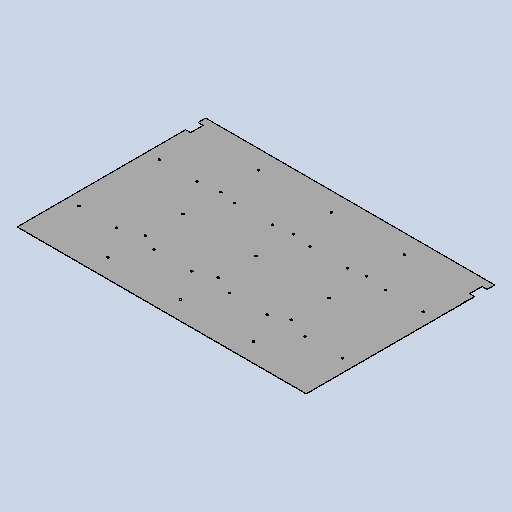
# Autodesk Inventor part: GnG L.4 floor sheet
Saved by Autodesk Inventor 2025.3 (Build 293356030, 356C)
## iProperties
Created: 2025-10-28
Part Number: GnG L.4 floor sheet
Material: Stainless Steel
Document SubType Name: Sheet Metal
Designer: admin
Mass: 82475.1 g
Surface Area: 69006.6 cm^2
Volume: 10309.4 cm^3
Density: 8 g/cm^3
Sheet Metal Rule: AISI304 3mm Die 32
Sheet Metal Width: 2300,000 mm
Sheet Metal Length: 1500,000 mm
Sheet Metal Area: 3450000,000 mm^2
Appearance: Default
Stock Number: L 4
Flat Pattern Width: 230 cm
Flat Pattern Length: 150 cm
Flat Pattern Area: 34500 cm^2
Author: admin
Autodesk Inventor part; units mm, degrees
ref_plane "YZ Plane" through (0, 0, 0) normal (1, 0, 0) x (0, 1, 0)
ref_plane "XZ Plane" through (0, 0, 0) normal (0, 1, 0) x (-1, 0, 0)
ref_plane "XY Plane" through (0, 0, 0) normal (0, 0, 1) x (1, 0, 0)
sketch "Sketch1" plane through (0, 0, 0) normal (0, 0, 1) x (1, 0, 0)
  line L0 (0, 0) -> (-2300, 0)
  line L1 (-2300, 0) -> (-2300, -1500)
  line L2 (-2300, -1500) -> (0, -1500)
  line L3 (0, -1500) -> (0, 0)
  line L4 (0, 0) -> (-20, 0)
  line L5 (-20, 0) -> (-20, -20)
  line L6 (-20, -20) -> (0, -20)
  line L7 (0, -20) -> (0, 0)
  line L8 (0, -1500) -> (-20, -1500)
  line L9 (-20, -1500) -> (-20, -1480)
  line L10 (-20, -1480) -> (0, -1480)
  line L11 (0, -1480) -> (0, -1500)
  line L12 (-2300, 0) -> (-2280, 0)
  line L13 (-2280, 0) -> (-2280, -20)
  line L14 (-2280, -20) -> (-2300, -20)
  line L15 (-2300, -20) -> (-2300, 0)
  line L16 (-2300, -1500) -> (-2280, -1500)
  line L17 (-2280, -1500) -> (-2280, -1480)
  line L18 (-2280, -1480) -> (-2300, -1480)
  line L19 (-2300, -1480) -> (-2300, -1500)
  line L20 (-310, -1500) -> (-220, -1500)
  line L21 (-220, -1500) -> (-220, -1480)
  line L22 (-220, -1480) -> (-310, -1480)
  line L23 (-310, -1480) -> (-310, -1500)
  line L24 (-310, 0) -> (-220, 0)
  line L25 (-220, 0) -> (-220, -20)
  line L26 (-220, -20) -> (-310, -20)
  line L27 (-310, -20) -> (-310, 0)
  line L28 (-2300, -60) -> (-2260, -60)
  line L29 (-2260, -60) -> (-2260, -160)
  line L30 (-2260, -160) -> (-2300, -160)
  line L31 (-2300, -160) -> (-2300, -60)
  line L32 (0, -60) -> (-40, -60)
  line L33 (-40, -60) -> (-40, -160)
  line L34 (-40, -160) -> (0, -160)
  line L35 (0, -160) -> (0, -60)
  point P0 (0, -20)
  point P1 (-20, 0)
  point P2 (-20, -1500)
  point P3 (0, -1480)
  point P4 (-220, -1500)
  point P5 (-220, 0)
  point P6 (-2280, 0)
  dimension "d22" = 2300
  dimension "d23" = 1500
  dimension "d24" = 20
  dimension "d25" = 20
  dimension "d28" = 90
  dimension "d29" = 200
  dimension "d70" = 40
  dimension "d71" = 100
  dimension "d72" = 60
  measures "d22" distance of L2.end L1.end
  measures "d23" distance of L1.end L0.end
  measures "d24" distance of L6.end L5.end
  measures "d25" distance of L5.end L4.end
  measures "d28" distance of L25.end L26.end
  measures "d29" distance between parallel lines of L5 L25
  measures "d70" distance of L29.end L30.end
  measures "d71" distance of L28.end L29.end
  measures "d72" distance between parallel lines of L28 L0
extrude "Plate1" add sketch "Sketch1" along normal blind 3 contours L3 L6 L5 L0 | L5 L6 L3 L32 L33 L34 L10 L9 L2 L21 L22 L23 L17 L18 L1 L30 L29 L28 L14 L13 L0 L27 L26 L25 | L25 L26 L27 L0 | L13 L14 L1 L0 | L3 L2 L9 L10 | L2 L23 L22 L21 | L18 L17 L2 L1
sketch "Sketch8" plane through (0, 0, 0) normal (0, 0, -1) x (-1, 0, 0)
  line L0 (0, -60) -> (0, 0) projected
  line L1 (2300, -1500) -> (0, -1500) projected
  line L2 (2300, 0) -> (2300, -60) projected
  line L3 (0, 0) -> (2300, 0) projected
  line L4 (0, -204.8209) -> (2, -204.8209)
  line L5 (2, -204.8209) -> (2, -209.8209)
  line L6 (2, -209.8209) -> (0, -209.8209)
  line L7 (0, -209.8209) -> (0, -204.8209)
  circle A0 centre (0, -190.6018) radius 2.5
  line L8 (0, -1500) -> (0, 0) projected
  line L9 (0, -214.8209) -> (2, -214.8209)
  line L10 (2, -214.8209) -> (2, -219.8209)
  line L11 (2, -219.8209) -> (0, -219.8209)
  line L12 (0, -219.8209) -> (0, -214.8209)
  line L13 (0, -224.8209) -> (2, -224.8209)
  line L14 (2, -224.8209) -> (2, -229.8209)
  line L15 (2, -229.8209) -> (0, -229.8209)
  line L16 (0, -229.8209) -> (0, -224.8209)
  line L17 (0, -234.8209) -> (2, -234.8209)
  line L18 (2, -234.8209) -> (2, -239.8209)
  line L19 (2, -239.8209) -> (0, -239.8209)
  line L20 (0, -239.8209) -> (0, -234.8209)
  line L21 (0, -244.8209) -> (2, -244.8209)
  line L22 (2, -244.8209) -> (2, -249.8209)
  line L23 (2, -249.8209) -> (0, -249.8209)
  line L24 (0, -249.8209) -> (0, -244.8209)
  line L25 (0, -254.8209) -> (2, -254.8209)
  line L26 (2, -254.8209) -> (2, -259.8209)
  line L27 (2, -259.8209) -> (0, -259.8209)
  line L28 (0, -259.8209) -> (0, -254.8209)
  line L29 (0, -264.8209) -> (2, -264.8209)
  line L30 (2, -264.8209) -> (2, -269.8209)
  line L31 (2, -269.8209) -> (0, -269.8209)
  line L32 (0, -269.8209) -> (0, -264.8209)
  line L33 (0, -274.8209) -> (2, -274.8209)
  line L34 (2, -274.8209) -> (2, -279.8209)
  line L35 (2, -279.8209) -> (0, -279.8209)
  line L36 (0, -279.8209) -> (0, -274.8209)
  line L37 (0, -284.8209) -> (2, -284.8209)
  line L38 (2, -284.8209) -> (2, -289.8209)
  line L39 (2, -289.8209) -> (0, -289.8209)
  line L40 (0, -289.8209) -> (0, -284.8209)
  line L41 (40, -60) -> (0, -60) projected
  line L42 (40, -160) -> (40, -60) projected
  line L43 (0, -160) -> (40, -160) projected
  line L44 (0, -1500) -> (0, -160) projected
  line L45 (2300, -160) -> (2300, -1500) projected
  line L46 (2260, -160) -> (2300, -160) projected
  line L47 (2260, -60) -> (2260, -160) projected
  line L48 (2300, -60) -> (2260, -60) projected
  point P0 (0, -94.5188)
  point P1 (0, -99.5188)
  point P2 (0, -84.5188)
  point P3 (0, -89.5188)
  point P4 (0, -74.5188)
  point P5 (0, -79.5188)
  point P6 (0, -64.5188)
  point P7 (0, -69.5188)
  point P8 (0, -59.5188)
  point P9 (0, -244.8209)
  point P10 (0, -249.8209)
  point P11 (0, -234.8209)
  point P12 (0, -239.8209)
  point P13 (0, -224.8209)
  point P14 (0, -229.8209)
  point P15 (0, -214.8209)
  point P16 (0, -219.8209)
  dimension "d50" = 5
  dimension "d51" = 2
  dimension "d62" = 10
  dimension "d69" = 5
  constraints: 72 end point, 3 point on line, 2 parallel, 1 centre point, 1 horizontal, 1 perpendicular, 1 vertical, 64 other
  measures "d50" diameter of A0
  measures "d51" distance of L4.start L4.end
  measures "d62" distance of L4.start L9.start
  measures "d69" distance of L4.end L5.end
extrude "Cut3" cut sketch "Sketch8" against normal blind 3 contours L8 A0 | A0 L8 | L4 L5 L6 L7 | L9 L10 L11 L8 | L13 L14 L15 L8 | L17 L18 L19 L8 | L21 L22 L23 L8
sketch "Sketch9" plane through (0, 0, 0) normal (0, 0, -1) x (-1, 0, 0)
  line L0 (2, -229.8209) -> (0, -229.8209) construction
  line L1 (0, -234.8209) -> (0, -229.8209) construction
  line L2 (0, -234.8209) -> (2, -234.8209) construction
  line L3 (2, -234.8209) -> (2, -239.8209) construction
  line L4 (2, -239.8209) -> (0, -239.8209) construction
  line L5 (0, -244.8209) -> (0, -239.8209) construction
  line L6 (0, -244.8209) -> (2, -244.8209) construction
  line L7 (2, -244.8209) -> (2, -249.8209) construction
  line L8 (2, -249.8209) -> (0, -249.8209) construction
  line L9 (0, -1500) -> (0, -249.8209) construction
  line L10 (2300, -1500) -> (0, -1500) construction
  line L11 (2300, -160) -> (2300, -1500) construction
  line L12 (2260, -160) -> (2300, -160) construction
  line L13 (2260, -60) -> (2260, -160) construction
  line L14 (2300, -60) -> (2260, -60) construction
  line L15 (2300, 0) -> (2300, -60) construction
  line L16 (0, 0) -> (2300, 0) construction
  line L17 (0, -60) -> (0, 0) construction
  line L18 (40, -60) -> (0, -60) construction
  line L19 (40, -160) -> (40, -60) construction
  line L20 (0, -160) -> (40, -160) construction
  line L21 (0, -188.1018) -> (0, -160) construction
  arc A0 (0, -193.1018) -> (0, -188.1018) centre (0, -190.6018) ccw construction
  line L22 (0, -204.8209) -> (0, -193.1018) construction
  line L23 (0, -204.8209) -> (2, -204.8209) construction
  line L24 (2, -204.8209) -> (2, -209.8209) construction
  line L25 (2, -209.8209) -> (0, -209.8209) construction
  line L26 (0, -214.8209) -> (0, -209.8209) construction
  line L27 (0, -214.8209) -> (2, -214.8209) construction
  line L28 (2, -214.8209) -> (2, -219.8209) construction
  line L29 (2, -219.8209) -> (0, -219.8209) construction
  line L30 (0, -224.8209) -> (0, -219.8209) construction
  line L31 (0, -224.8209) -> (2, -224.8209) construction
  line L32 (2, -224.8209) -> (2, -229.8209) construction
  line L33 (2300, -470) -> (0, -470) construction
  line L34 (0, -1110) -> (2300, -1110) construction
  line L35 (1730, 0) -> (1730, -1500) construction
  line L36 (1150, 0) -> (1150, -1500) construction
  line L37 (570, 0) -> (570, -1500) construction
  circle A1 centre (2200, -470) radius 7.5
  circle A2 centre (2200, -1110) radius 7.5
  circle A3 centre (1730, -150) radius 7.5
  circle A4 centre (1150, -150) radius 7.5
  circle A5 centre (570, -150) radius 7.5
  circle A6 centre (1900, -470) radius 7.5
  circle A7 centre (1900, -1110) radius 7.5
  circle A8 centre (1600, -470) radius 7.5
  circle A9 centre (1600, -1110) radius 7.5
  circle A10 centre (1300, -470) radius 7.5
  circle A11 centre (1300, -1110) radius 7.5
  circle A12 centre (1000, -470) radius 7.5
  circle A13 centre (1000, -1110) radius 7.5
  circle A14 centre (700, -470) radius 7.5
  circle A15 centre (700, -1110) radius 7.5
  circle A16 centre (400, -470) radius 7.5
  circle A17 centre (400, -1110) radius 7.5
  circle A18 centre (100, -470) radius 7.5
  circle A19 centre (100, -1110) radius 7.5
  circle A20 centre (-200, -470) radius 7.5
  circle A21 centre (-200, -1110) radius 7.5
  circle A22 centre (-500, -470) radius 7.5
  circle A23 centre (-500, -1110) radius 7.5
  circle A24 centre (-800, -470) radius 7.5
  circle A25 centre (-800, -1110) radius 7.5
  circle A26 centre (1150, -450) radius 7.5
  circle A27 centre (1730, -450) radius 7.5
  circle A28 centre (570, -450) radius 7.5
  circle A29 centre (1150, -750) radius 7.5
  circle A30 centre (1730, -750) radius 7.5
  circle A31 centre (570, -750) radius 7.5
  circle A32 centre (1150, -1050) radius 7.5
  circle A33 centre (1730, -1050) radius 7.5
  circle A34 centre (570, -1050) radius 7.5
  circle A35 centre (1150, -1350) radius 7.5
  circle A36 centre (1730, -1350) radius 7.5
  circle A37 centre (570, -1350) radius 7.5
  circle A38 centre (1150, -1650) radius 7.5
  circle A39 centre (1730, -1650) radius 7.5
  circle A40 centre (570, -1650) radius 7.5
  circle A41 centre (1150, -1950) radius 7.5
  circle A42 centre (1730, -1950) radius 7.5
  circle A43 centre (570, -1950) radius 7.5
  dimension "d73" = 570
  dimension "d74" = 1150
  dimension "d75" = 1730
  dimension "d76" = 470
  dimension "d77" = 1110
  dimension "d78" = 150
  dimension "d79" = 100
  dimension "d80" = 15
  dimension "d83" = 300
  dimension "d90" = 300
  constraints: 43 centre point, 13 point on line, 10 end point, 5 perpendicular, 4 equal radius, 2 horizontal alignment, 2 midpoint, 1 horizontal, 1 vertical, 1 vertical alignment, 76 other
  measures "d73" distance between parallel lines of L35 L11
  measures "d74" distance between parallel lines of L11 L36
  measures "d75" distance between parallel lines of L11 L37
  measures "d76" distance between parallel lines of L33 L16
  measures "d77" distance between parallel lines of L34 L16
  measures "d78" distance from line of L16 A3.centre
  measures "d79" distance from line of L11 A1.centre
  measures "d80" diameter of A1
  measures "d83" distance of A1.centre A6.centre
  measures "d90" distance of A4.centre A26.centre
extrude "Cut4" cut sketch "Sketch9" against normal blind 3
equation "\"d24\" = d25"
equation "\"d67\" = Thickness"
equation "\"d95\" = Thickness"
equation "\"d2\" = Thickness"
equation "\"BendReliefWidth\" = Thickness"
equation "\"BendReliefDepth\" = 0.5 * Thickness"
equation "\"CornerReliefSize\" = 4 * Thickness"
equation "\"MinimumRemnant\" = 2 * Thickness"
equation "\"TransitionRadius\" = BendRadius"
equation "\"JacobiRadiusSize\" = BendRadius"
equation "\"GapSize\" = Thickness"
equation "\"Thickness\" = 3"
equation "\"BendRadius\" = 5"
body "Solid1"
